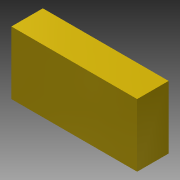
# Autodesk Inventor part: led
Saved by Autodesk Inventor 2015 (Build 190159000, 159)
## iProperties
Created: 2015-09-09
Part Number: led
Material: Generic
Document SubType Name: Modeling
Designer: david
Density: 1 g/cm^3
Appearance: Glossy - Gold
Author: david
Autodesk Inventor part; units mm, degrees
ref_plane "YZ Plane" through (0, 0, 0) normal (1, 0, 0) x (0, 1, 0)
ref_plane "XZ Plane" through (0, 0, 0) normal (0, 1, 0) x (-1, 0, 0)
ref_plane "XY Plane" through (0, 0, 0) normal (0, 0, 1) x (1, 0, 0)
sketch "Sketch1" plane through (0, 0, 0) normal (0, 1, 0) x (-1, 0, 0)
  line L0 (-1, 0.5) -> (1, 0.5)
  line L1 (1, 0.5) -> (1, -0.5)
  line L2 (1, -0.5) -> (-1, -0.5)
  line L3 (-1, -0.5) -> (-1, 0.5)
  line L4 (-1, 0.5) -> (1, -0.5) construction
  line L5 (1, 0.5) -> (-1, -0.5) construction
  point P0 (0, 0)
  dimension "d0" = 2
  dimension "d1" = 1
  constraints: 12 end point, 2 midpoint, 2 parallel, 1 horizontal, 1 perpendicular
  measures "d0" distance of L1.end L2.end
  measures "d1" distance of L0.end L1.end
extrude "Extrusion1" add sketch "Sketch1" along normal blind 0.5
body "Solid1"
